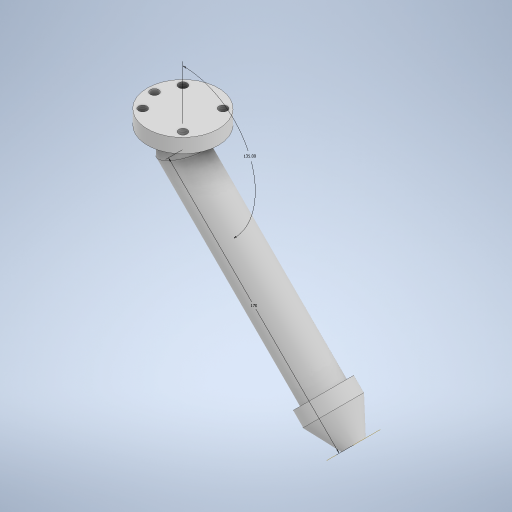
# Autodesk Inventor part: Herramienta total
Saved by Autodesk Inventor 2024 (Build 280153000, 153)
## iProperties
Created: 2024-02-19
Part Number: Herramienta total
Material: Genérico
Document SubType Name: Modeling
Designer: Juan David
Density: 1 g/cm^3
Appearance: Valor por defecto
Author: Juan David
Autodesk Inventor part; units mm, degrees
ref_plane "YZ Plane" through (0, 0, 0) normal (1, 0, 0) x (0, 1, 0)
ref_plane "XZ Plane" through (0, 0, 0) normal (0, 1, 0) x (-1, 0, 0)
ref_plane "XY Plane" through (0, 0, 0) normal (0, 0, 1) x (1, 0, 0)
sketch "Boceto1" plane through (0, 0, 0) normal (0, 1, 0) x (-1, 0, 0)
  circle A0 centre (0, 0) radius 25
  circle A1 centre (0, 0) radius 20
  line L0 (0, 0) -> (25, 0)
  line L1 (0, 0) -> (17.67767, -17.67767)
  line L2 (0, 0) -> (25, 0) construction
  line L3 (0, 0) -> (17.67767, 17.67767)
  line L4 (0, 0) -> (25, 0) construction
  line L5 (0, 0) -> (-17.67767, -17.67767)
  line L6 (0, 0) -> (-17.67767, 17.67767)
  circle A2 centre (20, 0) radius 3
  circle A3 centre (14.142136, -14.142136) radius 3
  circle A4 centre (14.142136, 14.142136) radius 3
  circle A5 centre (-14.142136, 14.142136) radius 3
  circle A6 centre (-14.142136, -14.142136) radius 3
  point P0 (16.098382, 11.867691)
  point P1 (11.867691, 16.098382)
  dimension "d0" = 50
  dimension "d1" = 40
  dimension "d2" = 45
  dimension "d3" = 45
  dimension "d4" = 6
  dimension "d5" = 6
  dimension "d6" = 6
  dimension "d7" = 6
  dimension "d8" = 6
  constraints: 14 end point, 10 point on circle, 7 centre point, 7 point on line, 3 horizontal, 2 coincident, 2 equal length
  measures "d0" diameter of A0
  measures "d1" diameter of A1
  measures "d2" angle of L1 L2
  measures "d3" angle of L4 L3
  measures "d4" diameter of A2
  measures "d5" diameter of A3
  measures "d6" diameter of A4
  measures "d7" diameter of A5
  measures "d8" diameter of A6
extrude "Extrusión1" add sketch "Boceto1" along normal blind 10 contours L0 A2 A1 A4 L3 A0 | A0 L1 A3 A1 A2 L0 | L3 A4 A1 A5 L6 A0 | A0 L5 A6 A1 A3 L1 | L6 A5 A1 A6 L5 A0 | A2 L0 L3 A4 A1 | A1 A3 L1 L0 A2 | A4 L3 L6 A5 A1 | A1 A6 L5 L1 A3 | A5 L6 L5 A6 A1
thread "Rosca1"
thread "Rosca2"
thread "Rosca3"
thread "Rosca4"
sketch "Boceto7" plane through (0, 0, 0) normal (0, 0, 1) x (1, 0, 0)
  line L0 (0, 0) -> (0, -15)
  line L1 (0, -15) -> (98.994949, -113.994949)
  dimension "d31" = 15
  dimension "d32" = 140
  dimension "d33" = 135
  constraints: 4 end point, 1 vertical
  measures "d31" distance of L0.start L0.end
  measures "d32" distance of L0.end L1.end
  measures "d33" angle of L1 L0
sketch "Boceto8" plane through (0, 0, 0) normal (0, -1, 0) x (1, 0, 0)
  circle A0 centre (0, 0) radius 13.5
  dimension "d34" = 27
  constraints: 1 centre point, 1 coincident
  measures "d34" diameter of A0
sweep "Barrido1" add profiles "Boceto8" path "Boceto7"
sketch "Boceto13" plane through (0, 0, 0) normal (0, 0, 1) x (1, 0, 0)
  line L0 (0, 0) -> (0, -15)
  line L1 (0, -15) -> (120.208153, -135.208153)
  dimension "d48" = 170
  dimension "d49" = 135
  constraints: 4 end point, 1 vertical
  measures "d48" distance of L0.end L1.end
  measures "d49" angle of L1 L0
sketch "Boceto14" plane through (98.994949, -113.994949, 0) normal (0.7071068, -0.7071068, 0) x (-0.7071068, -0.7071068, 0)
  ellipse E0 centre (-17.67767, 0) end of major axis (-17.67767, -25) minor radius 17.67767
  circle A0 centre (0, 0) radius 17.5
  point P0 (-10.606602, 0)
  dimension "d50" = 35
  constraints: 1 centre point, 1 horizontal alignment, 1 other
  measures "d50" diameter of A0
extrude "Extrusión9" add sketch "Boceto14" along normal blind 10 contours A0 E0 | E0 A0 picked at (-5.916701, -1.209366) picked at (5.555683, -1.849173)
ref_plane "Plano de trabajo1" through (120.208153, -135.208153, 0) normal (0.7071068, -0.7071068, 0) x (0.7071068, 0.7071068, 0)
sketch "Boceto16" plane through (120.208153, -135.208153, 0) normal (0.7071068, -0.7071068, 0) x (0.7071068, 0.7071068, 0)
  ellipse E0 centre (17.67767, 0) end of major axis (17.67767, 25) minor radius 17.67767
  circle A0 centre (0, 0) radius 7
  point P0 (10.606602, 0)
  dimension "d58" = 14
  constraints: 1 centre point, 1 horizontal alignment, 1 other
  measures "d58" diameter of A0
sketch "Boceto16 outline for Extrusión10" plane through (120.208153, -135.208153, 0) normal (0.7071068, -0.7071068, 0) x (0.7071068, 0.7071068, 0)
  circle A0 centre (0, 0) radius 7
extrude "Extrusión10" add sketch "Boceto16 outline for Extrusión10" against normal blind 20 draft 28
